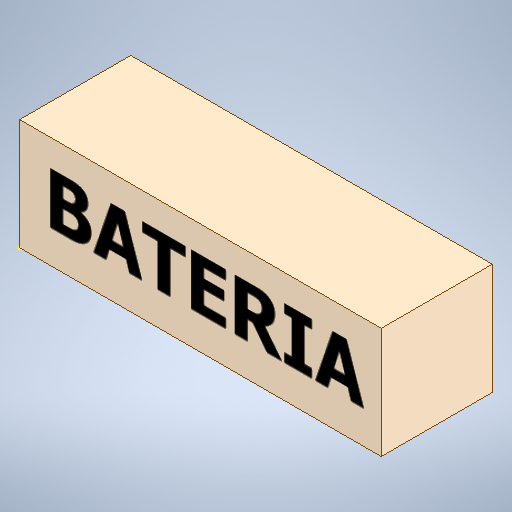
# Autodesk Inventor part: BATERIA
Saved by Autodesk Inventor 2025.3 (Build 293356030, 356C)
## iProperties
Created: 2025-07-08
Part Number: BATERIA
Material: Generic
Document SubType Name: Modeling
Designer: jv
Density: 1 g/cm^3
Appearance: Default(1)
Author: jv
Autodesk Inventor part; units mm, degrees
ref_plane "YZ Plane" through (0, 0, 0) normal (1, 0, 0) x (0, 1, 0)
ref_plane "XZ Plane" through (0, 0, 0) normal (0, 1, 0) x (-1, 0, 0)
ref_plane "XY Plane" through (0, 0, 0) normal (0, 0, 1) x (1, 0, 0)
sketch "Sketch1" plane through (0, 0, 0) normal (0, 0, 1) x (1, 0, 0)
  line L0 (0, 43) -> (140, 43)
  line L1 (140, 43) -> (140, 0)
  line L2 (140, 0) -> (0, 0)
  line L3 (0, 0) -> (0, 43)
  dimension "d0" = 140
  dimension "d1" = 43
  constraints: 8 end point, 2 parallel, 1 coincident, 1 horizontal, 1 perpendicular
  measures "d0" distance of L1.end L2.end
  measures "d1" distance of L0.end L1.end
extrude "Extrusion1" add sketch "Sketch1" along normal blind 43
sketch "Sketch2" plane through (0, 0, 43) normal (0, 0, 1) x (1, 0, 0)
  line L0 (18.8991, 36.6866) -> (124.2897, 36.6866) construction
  line L1 (124.2897, 36.6866) -> (124.2897, 8.6714) construction
  line L2 (124.2897, 8.6714) -> (18.8991, 8.6714) construction
  line L3 (18.8991, 8.6714) -> (18.8991, 36.6866) construction
  point P0 (0, 0)
  constraints: 2 other
body "Solid1"
